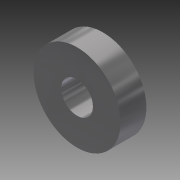
# Autodesk Inventor part: Big Bearing
Saved by Autodesk Inventor 2014 (Build 180170000, 170)
## iProperties
Created: 2015-02-07
Part Number: Big Bearing
Material: Steel, Carbon
Document SubType Name: Modeling
Designer: Spooner
Density: 7.87 g/cm^3
Appearance: Semi-Polished
Author: Spooner
Autodesk Inventor part; units mm, degrees
sketch "Sketch1" plane through (0, 0, 0) normal (0, 0, 1) x (1, 0, 0)
  circle A0 centre (0, 0) radius 8.5725
  circle A1 centre (0, 0) radius 23.495
  dimension "d0" = 46.99
  dimension "d1" = 17.145
  constraints: 2 centre point, 2 coincident
  measures "d0" diameter of A1
  measures "d1" diameter of A0
extrude "Extrusion1" add sketch "Sketch1" along normal blind 13.97
ref_plane "Work Plane1" through (0, 0, 6.985) normal (0, 0, 1) x (1, 0, 0)
ref_plane "Work Plane2" through (0, 0, 0) normal (0, 1, 0) x (0, 0, 1)
ref_plane "Work Plane3" through (0, 0, 0) normal (1, 0, 0) x (0, 0, 1)
body "Solid1"
